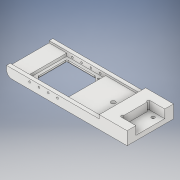
# Autodesk Inventor part: TNS_Greiferbacke_MA_Jun_T1
Saved by Autodesk Inventor 2017 (Build 210142000, 142)
## iProperties
Created: 2018-03-13
Part Number: TNS_Greiferbacke_MA_Jun_T1
Material: Generic
Document SubType Name: Modeling
Designer: uoehq
Density: 1 g/cm^3
Appearance: Snow
Author: uoehq
Autodesk Inventor part; units mm, degrees
ref_plane "YZ Plane" through (0, 0, 0) normal (1, 0, 0) x (0, 1, 0)
ref_plane "XZ Plane" through (0, 0, 0) normal (0, 1, 0) x (-1, 0, 0)
ref_plane "XY Plane" through (0, 0, 0) normal (0, 0, 1) x (1, 0, 0)
sketch "unten" plane through (0, 0, 0) normal (0, 0, 1) x (1, 0, 0)
  line L0 (0, 0) -> (130, 0)
  line L1 (130, 0) -> (130, -50)
  line L2 (130, -50) -> (0, -50)
  line L3 (0, -50) -> (0, 0)
  line L4 (23.5, -7) -> (52.1715, -7)
  line L5 (58, -12.8285) -> (58, -41.5)
  line L6 (27.8285, -43) -> (56.5, -43)
  line L7 (22, -8.5) -> (22, -37.1715)
  arc A0 (23.5, -7) -> (22, -8.5) centre (23.5, -8.5) ccw
  circle A1 centre (23, -42) radius 1
  circle A2 centre (57, -8) radius 1
  arc A3 (56.5, -43) -> (58, -41.5) centre (56.5, -41.5) ccw
  line L8 (61.9906, -8.5458) -> (71.0184, -8.5458) construction
  line L9 (53.5857, -7.5858) -> (57.4142, -11.4143)
  line L10 (57.2091, -11.2092) -> (62.6234, -11.2092) construction
  arc A4 (58, -12.8285) -> (57.4142, -11.4143) centre (56, -12.8285) ccw
  arc A5 (53.5857, -7.5858) -> (52.1715, -7) centre (52.1715, -9) ccw
  line L11 (22.5858, -38.5857) -> (26.4143, -42.4142)
  line L12 (26.3083, -42.3082) -> (31.7226, -42.3082) construction
  arc A6 (22, -37.1715) -> (22.5858, -38.5857) centre (24, -37.1715) ccw
  arc A7 (26.4143, -42.4142) -> (27.8285, -43) centre (27.8285, -41) ccw
  line L13 (130, -9.5) -> (130, -40.5)
  line L14 (130, -50) -> (130, 0)
  line L15 (130, 0) -> (130, -50)
  point P0 (33.5, -8.5)
  dimension "d0" = 130
  dimension "d1" = 50
  dimension "d15" = 1.5
  dimension "d18" = 2
  dimension "d21" = 2
  dimension "d24" = 1.5
  dimension "d29" = 45
  dimension "d31" = 2
  dimension "d32" = 45
  dimension "d34" = 2
  dimension "d51" = 7
  dimension "d52" = 7
  dimension "d53" = 36
  dimension "d55" = 8
  dimension "d56" = 1
  dimension "d57" = 1
  dimension "d58" = 1
  dimension "d59" = 2.1214
  dimension "d60" = 22
  dimension "d61" = 1.5
  dimension "d62" = 1.5
  dimension "d63" = 2.1214
  dimension "d64" = 1.5
  dimension "d65" = 1.5
  constraints: 32 end point, 12 point on circle, 8 centre point, 8 tangent, 6 horizontal, 4 point on line, 2 coincident, 2 collinear, 2 equal length, 2 equal radius, 2 parallel, 2 vertical, 1 perpendicular
  measures "d0" distance of L0.start L0.end
  measures "d1" distance of L0.end L1.end
  measures "d15" radius of A0
  measures "d18" diameter of A1
  measures "d21" diameter of A2
  measures "d24" radius of A3
  measures "d29" angle of L9 L10
  measures "d31" radius of A4
  measures "d32" angle of L11 L12
  measures "d34" radius of A6
  measures "d51" distance between parallel lines of L0 L4
  measures "d52" distance between parallel lines of L2 L6
  measures "d53" distance between parallel lines of L5 L7
  measures "d55" distance from line of L0 A2.centre
  measures "d56" distance from line of L5 A2.centre
  measures "d57" distance from line of L7 A1.centre
  measures "d58" distance from line of L6 A1.centre
  measures "d59" distance from line of A1.centre L11
  measures "d60" distance between parallel lines of L3 L7
  measures "d61" distance from line of L7 A0.centre
  measures "d62" distance from line of L4 A0.centre
  measures "d63" distance from line of A2.centre L9
  measures "d64" distance from line of L5 A3.centre
  measures "d65" distance from line of A3.centre L6
extrude "Extrusion1" add sketch "unten" along normal blind 10
sketch "Sketch2" plane through (0, 0, 10) normal (0, 0, 1) x (1, 0, 0)
  line L0 (114, -9.5) -> (130, -9.5)
  line L1 (130, -50) -> (130, 0) projected
  line L2 (130, 0) -> (0, 0) projected
  line L3 (130, -9.5) -> (130, 0)
  line L4 (130, 0) -> (0, 0) projected
  line L5 (130, 0) -> (100, 0)
  line L6 (100, 0) -> (100, -50)
  line L7 (0, -50) -> (130, -50) projected
  line L8 (130, -50) -> (130, -40.5)
  line L9 (130, -40.5) -> (114, -40.5)
  line L10 (114, -12.5) -> (114, -37.5)
  arc A0 (114, -9.5) -> (114, -12.5) centre (114, -11) ccw
  arc A1 (114, -37.5) -> (114, -40.5) centre (114, -39) ccw
  dimension "d69" = 16
  dimension "d70" = 9.5
  dimension "d71" = 30
  dimension "d72" = 9.5
  dimension "d73" = 16
  dimension "d74" = 16
  dimension "d75" = 16
  dimension "d77" = 1.5
  dimension "d78" = 3
  dimension "d80" = 1.5
  constraints: 14 end point, 4 point on circle, 4 point on line, 2 centre point, 2 coincident, 2 perpendicular, 1 collinear, 1 horizontal, 1 vertical
  measures "d69" distance of L0.start L0.end
  measures "d70" distance between parallel lines of L2 L0
  measures "d71" distance of L1.end L5.end
  measures "d72" distance of L1.start L8.end
  measures "d73" distance of L8.end L9.end
  measures "d74" distance from line of L1 point (114, -11)
  measures "d75" distance from line of L1 point (114, -39)
  measures "d77" distance of L0.start point (114, -11)
  measures "d78" distance of L0.start L10.start
  measures "d80" distance from line of L9 A1.centre
extrude "Extrusion2" add sketch "Sketch2" along normal blind 4 contours A0 L10 A1 L9 L1 L7 L6 L2 L0
sketch "Sketch3" plane through (0, 0, 10) normal (0, 0, 1) x (1, 0, 0)
  line L0 (100, -50) -> (100, 0) projected
  line L1 (0, -4) -> (100, -4)
  line L2 (100, -4) -> (100, -46)
  line L3 (100, -46) -> (0, -46)
  line L4 (0, -46) -> (0, -4)
  line L5 (100, 0) -> (0, 0) projected
  line L6 (0, -50) -> (100, -50) projected
  dimension "d83" = 4
  dimension "d84" = 4
  constraints: 8 end point, 2 parallel, 1 horizontal, 1 perpendicular, 1 point on line
  measures "d83" distance between parallel lines of L5 L1
  measures "d84" distance between parallel lines of L6 L3
extrude "Extrusion3" cut sketch "Sketch3" against normal blind 2
sketch "Sketch4" plane through (0, 0, 8) normal (0, 0, 1) x (1, 0, 0)
  line L0 (61, -4) -> (19, -4)
  line L1 (19, -4) -> (19, -46)
  line L2 (19, -46) -> (61, -46)
  line L3 (61, -46) -> (61, -4)
  line L4 (22, -8.5) -> (22, -37.1715) projected
  line L5 (27.8285, -43) -> (56.5, -43) projected
  point P0 (0, 0)
  dimension "d87" = 42
  dimension "d88" = 42
  dimension "d89" = 3
  dimension "d90" = 3
  constraints: 8 end point, 2 parallel, 1 horizontal, 1 perpendicular
  measures "d87" distance between parallel lines of L1 L3
  measures "d88" distance between parallel lines of L0 L2
  measures "d89" distance between parallel lines of L1 L4
  measures "d90" distance between parallel lines of L2 L5
extrude "Extrusion4" cut sketch "Sketch4" against normal blind 3
sketch "Sketch5" plane through (0, 0, 0) normal (0, 0, -1) x (-1, 0, 0)
  line L0 (-19, -46) -> (-19, -4) projected
  line L1 (-61, -4) -> (-61, -46) projected
  line L2 (-19, -46) -> (-61, -46)
  line L3 (-61, -46) -> (-61, -4)
  line L4 (-61, -4) -> (-19, -4)
  line L5 (-19, -4) -> (-19, -46)
  point P0 (0, 0)
  constraints: 8 end point, 2 parallel, 1 horizontal, 1 perpendicular
extrude "Extrusion5" cut sketch "Sketch5" against normal blind 3.4
fillet "Fillet1" radius 6 1 edges at (0, -25, 0)
sketch "Sketch6" plane through (0, 0, 0) normal (0, 0, -1) x (-1, 0, 0)
  line L0 (-6, -50) -> (-130, -50) projected
  line L1 (-130, 0) -> (-6, 0) projected
  line L2 (-130, -50) -> (-130, 0) projected
  point P0 (0, 0)
  point P1 (-122.5, -35.5)
  point P2 (-122.5, -14.5)
  dimension "d96" = 14.5
  dimension "d97" = 14.5
  dimension "d98" = 7.5
  dimension "d99" = 7.5
  measures "d96" distance from line of L0 point (-122.5, -35.5)
  measures "d97" distance from line of L1 point (-122.5, -14.5)
  measures "d98" distance from line of L2 point (-122.5, -35.5)
  measures "d99" distance from line of L2 point (-122.5, -14.5)
hole "Hole1" at (122.5, -35.5, 0) at (122.5, -14.5, 0) direction (0, 0, 1) diameter 3.5 end through all counterbore diameter 6 counterbore depth 3
sketch "Sketch7" plane through (0, 0, 0) normal (0, 0, -1) x (-1, 0, 0)
  line L0 (-130, 0) -> (-6, 0) projected
  line L1 (-100, -4) -> (-100, -46) projected
  point P0 (0, 0)
  point P1 (-90, -25)
  dimension "d119" = 25
  dimension "d120" = 10
  measures "d119" distance from line of L0 point (-90, -25)
  measures "d120" distance from line of L1 point (-90, -25)
hole "Hole2" at (90, -25, 0) direction (0, 0, 1) diameter 4.5 end through all counterbore diameter 8 counterbore depth 3
hole "Hole4" at (25, -50, 7) direction (0, 1, 0) diameter 2 end through all
pattern_linear "Rectangular Pattern1" count 4 spacing 10 along (1, 0, 0) of "Hole4"
sketch "Sketch10" plane through (0, 0, 10) normal (0, 0, 1) x (1, 0, 0)
  line L0 (130, -9.5) -> (114, -9.5) projected
  line L1 (130, -9.5) -> (114, -9.5)
  arc A0 (114, -9.5) -> (114, -12.5) centre (114, -11) ccw projected
  arc A1 (114, -12.5) -> (114, -12.5) centre (114, -11) ccw
  arc A2 (114, -37.5) -> (114, -40.5) centre (114, -39) ccw projected
  line L2 (114, -12.5) -> (114, -37.5)
  arc A3 (114, -37.5) -> (114, -40.5) centre (114, -39) ccw
  line L3 (114, -40.5) -> (130, -40.5) projected
  line L4 (114, -40.5) -> (130, -40.5)
  line L5 (130, -50) -> (130, 0) projected
  line L6 (130, -40.5) -> (130, -9.5) projected
  line L7 (130, -9.5) -> (130, -40.5)
  point P0 (0, 0)
  constraints: 8 end point, 4 point on circle, 2 centre point, 2 coincident, 2 vertical, 1 collinear, 1 horizontal, 1 point on line
extrude "Extrusion6" cut sketch "Sketch10" against normal blind 5
body "Solid1"
